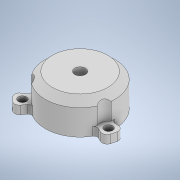
# Autodesk Inventor part: Knob
Saved by Autodesk Inventor 2022 (Build 260153000, 153)
## iProperties
Created: 2022-04-06
Part Number: Knob
Material: Generic
Document SubType Name: Modeling
Designer: awp
Density: 1 g/cm^3
Appearance: Default
Author: awp
Autodesk Inventor part; units mm, degrees
ref_plane "YZ Plane" through (0, 0, 0) normal (1, 0, 0) x (0, 1, 0)
ref_plane "XZ Plane" through (0, 0, 0) normal (0, 1, 0) x (-1, 0, 0)
ref_plane "XY Plane" through (0, 0, 0) normal (0, 0, 1) x (1, 0, 0)
sketch "Sketch1" plane through (0, 0, 0) normal (0, 1, 0) x (-1, 0, 0)
  circle A0 centre (0, 0) radius 2
  circle A1 centre (0, 0) radius 12.7
  dimension "d0" = 4
  dimension "d1" = 25.4
  constraints: 2 centre point, 2 coincident
  measures "d0" diameter of A0
  measures "d1" diameter of A1
extrude "Extrusion1" add sketch "Sketch1" along normal blind 3
sketch "Sketch3" plane through (0, 0, 0) normal (0, -1, 0) x (1, 0, 0)
  circle A0 centre (0, 0) radius 11.1125
  circle A1 centre (0, 0) radius 12.7 projected
  circle A2 centre (0, 0) radius 2 projected
  circle A3 centre (0, 0) radius 12.7 projected
  circle A4 centre (0, 0) radius 2 projected
  circle A5 centre (0, 0) radius 12.7
  dimension "d14" = 22.225
  constraints: 2 centre point, 2 coincident, 1 concentric
  measures "d14" diameter of A0
extrude "Extrusion3" add sketch "Sketch3" along normal blind 8.858 contours A1
sketch "Sketch4" plane through (0, 0, 0) normal (0, -1, 0) x (1, 0, 0)
  circle A0 centre (0, 0) radius 2 projected
  circle A1 centre (0, 0) radius 2 projected
  line L0 (-1.9732, -0.3262) -> (-3.4732, -0.3262)
  line L1 (-3.4732, -0.3262) -> (-1.9933, -0.3262)
  line L2 (-1.9933, -0.3262) -> (-1.9933, 7.2938)
  line L3 (-1.9933, 7.2938) -> (-3.4732, 7.2938)
  line L4 (-3.4732, 7.2938) -> (-3.4732, -0.3262)
  line L5 (-3.4732, 7.2938) -> (-4.7432, 7.2938)
  line L6 (-4.7432, 7.2938) -> (-4.7432, 3.4838)
  line L7 (-4.7432, 3.4838) -> (-3.4732, 3.4838)
  line L8 (-3.4732, 3.4838) -> (-3.4732, 7.2938)
  line L9 (-1.9933, 7.2938) -> (-0.7233, 7.2938)
  line L10 (-0.7233, 7.2938) -> (-0.7233, 3.4838)
  line L11 (-0.7233, 3.4838) -> (-1.9933, 3.4838)
  line L12 (-1.9933, 3.4838) -> (-1.9933, 7.2938)
  line L13 (-3.4732, -0.3262) -> (-1.9933, -0.3262)
  line L14 (-1.9933, -0.3262) -> (-1.9933, -7.3112)
  line L15 (-1.9933, -7.3112) -> (-3.4732, -7.3112)
  line L16 (-3.4732, -7.3112) -> (-3.4732, -0.3262)
  line L17 (-3.4732, -7.3112) -> (-4.7432, -7.3112)
  line L18 (-4.7432, -7.3112) -> (-4.7432, -3.5012)
  line L19 (-4.7432, -3.5012) -> (-3.4732, -3.5012)
  line L20 (-3.4732, -3.5012) -> (-3.4732, -7.3112)
  line L21 (-1.9933, -7.3112) -> (-0.7233, -7.3112)
  line L22 (-0.7233, -7.3112) -> (-0.7233, -3.5012)
  line L23 (-0.7233, -3.5012) -> (-1.9933, -3.5012)
  line L24 (-1.9933, -3.5012) -> (-1.9933, -7.3112)
  line L25 (-3.4732, -7.3112) -> (-4.7432, -6.0412)
  line L26 (-3.4732, -7.3112) -> (-1.6772, -7.3112) construction
  point P0 (-1.9933, 3.4838)
  point P1 (-3.4732, 3.4838)
  point P2 (-3.4732, -3.5012)
  point P3 (-1.9933, -3.5012)
  dimension "d17" = 1.5
  dimension "d18" = 7.62
  dimension "d19" = 1.27
  dimension "d20" = 3.81
  dimension "d21" = 1.27
  dimension "d22" = 3.81
  dimension "d37" = 6.985
  dimension "d38" = 1.27
  dimension "d39" = 3.81
  dimension "d40" = 1.27
  dimension "d41" = 135
  constraints: 54 end point, 12 parallel, 8 horizontal, 6 perpendicular, 2 point on line, 1 equal length, 2 other
  measures "d17" distance of L0.start L0.end
  measures "d18" distance of L2.end L1.end
  measures "d19" distance of L7.end L6.end
  measures "d20" distance of L6.end L5.end
  measures "d21" distance of L10.end L11.end
  measures "d22" distance of L9.end L10.end
  measures "d37" distance of L13.end L14.end
  measures "d38" distance of L18.end L19.end
  measures "d39" distance of L17.end L18.end
  measures "d40" distance of L23.end L22.end
  measures "d41" angle of L26 L25
extrude "Extrusion4" add sketch "Sketch4" along normal blind 2 contours L23 L22 L21 L14 | L16 L25 L18 L19
sketch "Sketch5" plane through (0, 3, 0) normal (0, 1, 0) x (1, 0, 0)
  circle A0 centre (0, 0) radius 12.7 projected
  circle A1 centre (0, 0) radius 2 projected
  circle A2 centre (0, 0) radius 12.7 projected
  line L0 (0, 12.7) -> (0, 14.605)
  line L1 (0, 14.605) -> (2.0758, 12.5292)
  line L2 (0, 14.605) -> (-2.0758, 12.5292)
  line L3 (0, 14.605) -> (2.9356, 14.605) construction
  line L4 (-4.5132, 13.8902) -> (-1.8975, 12.5574)
  line L5 (-3.9245, 12.0784) -> (-4.5132, 13.8902)
  line L6 (-4.5132, 13.8902) -> (-5.8459, 11.2745)
  line L7 (-8.5846, 11.8157) -> (-5.6851, 11.3565)
  line L8 (-7.4649, 10.2745) -> (-8.5846, 11.8157)
  line L9 (-8.5846, 11.8157) -> (-9.0438, 8.9162)
  line L10 (-11.8157, 8.5846) -> (-8.9162, 9.0438)
  line L11 (-10.2745, 7.4649) -> (-11.8157, 8.5846)
  line L12 (-11.8157, 8.5846) -> (-11.3565, 5.6851)
  line L13 (-13.8902, 4.5132) -> (-11.2745, 5.8459)
  line L14 (-12.0784, 3.9245) -> (-13.8902, 4.5132)
  line L15 (-13.8902, 4.5132) -> (-12.5574, 1.8975)
  line L16 (-14.605, 0) -> (-12.5292, 2.0758)
  line L17 (-12.7, 0) -> (-14.605, 0)
  line L18 (-14.605, 0) -> (-12.5292, -2.0758)
  line L19 (-13.8902, -4.5132) -> (-12.5574, -1.8975)
  line L20 (-12.0784, -3.9245) -> (-13.8902, -4.5132)
  line L21 (-13.8902, -4.5132) -> (-11.2745, -5.8459)
  line L22 (-11.8157, -8.5846) -> (-11.3565, -5.6851)
  line L23 (-10.2745, -7.4649) -> (-11.8157, -8.5846)
  line L24 (-11.8157, -8.5846) -> (-8.9162, -9.0438)
  line L25 (-8.5846, -11.8157) -> (-9.0438, -8.9162)
  line L26 (-7.4649, -10.2745) -> (-8.5846, -11.8157)
  line L27 (-8.5846, -11.8157) -> (-5.6851, -11.3565)
  line L28 (-4.5132, -13.8902) -> (-5.8459, -11.2745)
  line L29 (-3.9245, -12.0784) -> (-4.5132, -13.8902)
  line L30 (-4.5132, -13.8902) -> (-1.8975, -12.5574)
  line L31 (0, -14.605) -> (-2.0758, -12.5292)
  line L32 (0, -12.7) -> (0, -14.605)
  line L33 (0, -14.605) -> (2.0758, -12.5292)
  line L34 (4.5132, -13.8902) -> (1.8975, -12.5574)
  line L35 (3.9245, -12.0784) -> (4.5132, -13.8902)
  line L36 (4.5132, -13.8902) -> (5.8459, -11.2745)
  line L37 (8.5846, -11.8157) -> (5.6851, -11.3565)
  line L38 (7.4649, -10.2745) -> (8.5846, -11.8157)
  line L39 (8.5846, -11.8157) -> (9.0438, -8.9162)
  line L40 (11.8157, -8.5846) -> (8.9162, -9.0438)
  line L41 (10.2745, -7.4649) -> (11.8157, -8.5846)
  line L42 (11.8157, -8.5846) -> (11.3565, -5.6851)
  line L43 (13.8902, -4.5132) -> (11.2745, -5.8459)
  line L44 (12.0784, -3.9245) -> (13.8902, -4.5132)
  line L45 (13.8902, -4.5132) -> (12.5574, -1.8975)
  line L46 (14.605, 0) -> (12.5292, -2.0758)
  line L47 (12.7, 0) -> (14.605, 0)
  line L48 (14.605, 0) -> (12.5292, 2.0758)
  line L49 (13.8902, 4.5132) -> (12.5574, 1.8975)
  line L50 (12.0784, 3.9245) -> (13.8902, 4.5132)
  line L51 (13.8902, 4.5132) -> (11.2745, 5.8459)
  line L52 (11.8157, 8.5846) -> (11.3565, 5.6851)
  line L53 (10.2745, 7.4649) -> (11.8157, 8.5846)
  line L54 (11.8157, 8.5846) -> (8.9162, 9.0438)
  line L55 (8.5846, 11.8157) -> (9.0438, 8.9162)
  line L56 (7.4649, 10.2745) -> (8.5846, 11.8157)
  line L57 (8.5846, 11.8157) -> (5.6851, 11.3565)
  line L58 (4.5132, 13.8902) -> (5.8459, 11.2745)
  line L59 (3.9245, 12.0784) -> (4.5132, 13.8902)
  line L60 (4.5132, 13.8902) -> (1.8975, 12.5574)
  point P0 (-1.9969, 12.6081)
  point P1 (-5.7953, 11.3739)
  point P2 (-9.0264, 9.0264)
  point P3 (-11.3739, 5.7953)
  point P4 (-12.6081, 1.9969)
  point P5 (-12.6081, -1.9969)
  point P6 (-11.3739, -5.7953)
  point P7 (-9.0264, -9.0264)
  point P8 (-5.7953, -11.3739)
  point P9 (-1.9969, -12.6081)
  point P10 (1.9969, -12.6081)
  point P11 (5.7953, -11.3739)
  point P12 (9.0264, -9.0264)
  point P13 (11.3739, -5.7953)
  point P14 (12.6081, -1.9969)
  point P15 (12.6081, 1.9969)
  point P16 (11.3739, 5.7953)
  point P17 (9.0264, 9.0264)
  point P18 (5.7953, 11.3739)
  point P19 (1.9969, 12.6081)
  dimension "d28" = 1.905
  dimension "d29" = 45
  dimension "d30" = 135
  dimension "d33" = 360
  constraints: 122 end point, 2 point on circle, 1 equal length, 1 horizontal, 1 vertical, 143 other
  measures "d28" distance of L0.start L0.end
  measures "d29" angle of L0 L1
  measures "d30" angle of L2 L3
extrude "Extrusion5" [suppressed]
fillet "Fillet1" [suppressed]
sketch "Sketch8" plane through (0, -8.858, 0) normal (0, -1, 0) x (1, 0, 0)
  circle A0 centre (13.4621, 6.4384) radius 1.5 projected
  line L0 (16.2108, 4.5139) -> (12.5404, 3.4919) projected
  arc A1 (12.5404, 3.4919) -> (10.5899, 7.5704) centre (0, 0) ccw projected
  line L1 (10.5899, 7.5704) -> (13.6893, 9.7861) projected
  arc A2 (16.2108, 4.5139) -> (13.6893, 9.7861) centre (0, 0) ccw projected
  circle A3 centre (-12.3435, 8.3856) radius 1.5 projected
  line L2 (-12.0145, 11.782) -> (-9.2943, 9.1144) projected
  arc A4 (-9.2943, 9.1144) -> (-11.851, 5.3859) centre (0, 0) ccw projected
  line L3 (-11.851, 5.3859) -> (-15.3196, 6.9623) projected
  arc A5 (-12.0145, 11.782) -> (-15.3196, 6.9623) centre (0, 0) ccw projected
  circle A6 centre (-1.2201, -14.8725) radius 1.5 projected
  line L4 (-4.1963, -16.2959) -> (-3.2462, -12.6063) projected
  arc A7 (-3.2462, -12.6063) -> (1.2612, -12.9563) centre (0, 0) ccw projected
  line L5 (1.2612, -12.9563) -> (1.6303, -16.7483) projected
  arc A8 (-4.1963, -16.2959) -> (1.6303, -16.7483) centre (0, 0) ccw projected
  circle A9 centre (0, 0) radius 12.7 projected
  line L6 (-4.1963, -16.2959) -> (-3.167, -12.2988)
  line L7 (1.6303, -16.7483) -> (1.2304, -12.6403)
  line L8 (16.2108, 4.5139) -> (12.2346, 3.4067)
  line L9 (13.6893, 9.7861) -> (10.3316, 7.3857)
  line L10 (-12.0145, 11.782) -> (-9.0676, 8.8921)
  line L11 (-15.3196, 6.9623) -> (-11.562, 5.2545)
  point P0 (10.5899, 7.5704)
  point P1 (-11.851, 5.3859)
  point P2 (1.2612, -12.9563)
  constraints: 12 end point, 6 point on circle, 2 point on line
extrude "Extrusion6" [suppressed]
fillet "Fillet2" [suppressed]
chamfer "Chamfer2" distance 2.54 angle 45 1 edges at (12.7, 3, 0)
sketch "Sketch9" plane through (0, 0, 0) normal (0, -1, 0) x (1, 0, 0)
  circle A0 centre (0, 0) radius 3
  circle A1 centre (0, 0) radius 4
  line L0 (-0.7233, -3.5012) -> (-1.9933, -3.5012) projected
  line L1 (-1.9933, -3.5012) -> (-1.9933, -7.3112) projected
  line L2 (-1.9933, -7.3112) -> (-0.7233, -7.3112) projected
  line L3 (-0.7233, -7.3112) -> (-0.7233, -3.5012) projected
  line L4 (-3.4732, -7.3112) -> (-3.4732, -3.5012) projected
  line L5 (-3.4732, -3.5012) -> (-4.7432, -3.5012) projected
  line L6 (-4.7432, -3.5012) -> (-4.7432, -6.0412) projected
  line L7 (-4.7432, -6.0412) -> (-3.4732, -7.3112) projected
  line L8 (-1.9933, -3.5012) -> (-1.9062, -2.3166)
  line L9 (-3.4732, -3.5012) -> (-4.7432, -3.5012) projected
  line L10 (-3.4732, -3.5012) -> (-3, 0)
  point P0 (-3.3046, -2.2538)
  point P1 (-1.991, -3.4693)
  dimension "d49" = 6
  dimension "d50" = 8
  constraints: 4 end point, 2 centre point, 2 coincident, 2 point on circle
  measures "d49" diameter of A0
  measures "d50" diameter of A1
extrude "Extrusion7" add sketch "Sketch9" along normal blind 6.35 contours A0 L10 A1 L3 L0 L8 | L0 L3 A1
sketch "Sketch10" plane through (0, 3, 0) normal (0, 1, 0) x (1, 0, 0)
  circle A0 centre (-12.3435, -8.3856) radius 1.5 projected
  circle A1 centre (-1.2201, 14.8725) radius 1.5 projected
  circle A2 centre (13.4621, -6.4384) radius 1.5 projected
  circle A3 centre (-12.3435, -8.3856) radius 3.175
  circle A4 centre (-1.2201, 14.8725) radius 3.175
  circle A5 centre (13.4621, -6.4384) radius 3.175
  point P0 (0, 0)
  dimension "d53" = 6.35
  dimension "d54" = 6.35
  dimension "d55" = 6.35
  constraints: 3 centre point, 3 coincident
  measures "d53" diameter of A3
  measures "d54" diameter of A4
  measures "d55" diameter of A5
extrude "Extrusion8" [suppressed]
fillet "Fillet3" [suppressed]
thicken "Thicken3" [suppressed]
thicken "Thicken4" [suppressed]
thicken "Thicken5" [suppressed]
sketch "Sketch11" plane through (0, 0, 0) normal (0, -1, 0) x (1, 0, 0)
  arc A0 (-0.7233, -3.9341) -> (-3.3046, -2.2538) centre (0, 0) ccw projected
  line L0 (-0.7233, -3.9341) -> (-0.7233, -7.3112) projected
  line L1 (-0.7233, -7.3112) -> (-1.9933, -7.3112) projected
  line L2 (-1.9933, -7.3112) -> (-1.9933, -3.5012) projected
  line L3 (-1.9933, -3.5012) -> (-1.9343, -3.5012) projected
  arc A1 (-1.991, -3.4693) -> (-1.9343, -3.5012) centre (0, 0) ccw projected
  line L4 (-1.991, -3.4693) -> (-1.9062, -2.3166) projected
  arc A2 (-1.9062, -2.3166) -> (-3, 0) centre (0, 0) ccw projected
  line L5 (-3, 0) -> (-3.3046, -2.2538) projected
  line L6 (-3.4732, -7.3112) -> (-4.7432, -6.0412) projected
  line L7 (-4.7432, -6.0412) -> (-4.7432, -3.5012) projected
  line L8 (-4.7432, -3.5012) -> (-3.4732, -3.5012) projected
  line L9 (-3.4732, -3.5012) -> (-3.4732, -7.3112) projected
  circle A3 centre (0, 0) radius 11.1125 projected
  circle A4 centre (0, 0) radius 2 projected
  line L10 (-3.3046, -2.2538) -> (-3.4732, -3.5012)
  line L11 (-1.9933, -7.3112) -> (-1.9933, -3.5012) projected
  line L12 (-1.9933, -7.3112) -> (-1.9933, -10.9323)
  line L13 (-3.4732, -7.3112) -> (-4.7432, -6.0412) projected
  line L14 (-3.4732, -7.3112) -> (-3.4732, -10.5558)
  circle A5 centre (0, 0) radius 11.1125 projected
  constraints: 6 end point, 1 collinear, 1 parallel, 1 point on circle, 2 other
extrude "Extrusion9" add sketch "Sketch11" along normal up to surface (2 mm away) contours A0 L10 L8 L7 L6 L14 A3 L12 L1 L0
sketch "Sketch12" plane through (0, -8.858, 0) normal (0, -1, 0) x (1, 0, 0)
  circle A0 centre (0, 0) radius 12.7 projected
  circle A1 centre (0, 0) radius 11.1125 projected
  arc A2 (15.5202, 1.4015) -> (17.1016, 3.5319) centre (15.3603, 3.1723) ccw
  arc A3 (17.1016, 3.5319) -> (16.5455, 5.5845) centre (0, 0) ccw
  arc A4 (16.5455, 5.5845) -> (14.1049, 6.6252) centre (14.8608, 5.0159) ccw
  line L0 (14.1049, 6.6252) -> (12.5922, 5.9147)
  arc A5 (10.9566, 6.422) -> (12.5922, 5.9147) centre (12.0523, 7.0642) ccw
  arc A6 (10.9566, 6.422) -> (-6.3392, 11.0047) centre (0, 0) ccw
  arc A7 (-8.0114, 11.3739) -> (-6.3392, 11.0047) centre (-6.9731, 12.1052) ccw
  line L1 (-8.0114, 11.3739) -> (-8.9738, 12.7402)
  arc A8 (-8.9738, 12.7402) -> (-11.6095, 13.0445) centre (-10.4274, 11.7163) ccw
  arc A9 (-11.6095, 13.0445) -> (-13.109, 11.5366) centre (0, 0) ccw
  arc A10 (-13.109, 11.5366) -> (-12.7901, 8.9026) centre (-11.7743, 10.3619) ccw
  line L2 (-12.7901, 8.9026) -> (-11.4184, 7.9479)
  arc A11 (-11.0399, 6.2777) -> (-11.4184, 7.9479) centre (-12.1439, 6.9055) ccw
  arc A12 (-11.0399, 6.2777) -> (-6.3608, -10.9923) centre (0, 0) ccw
  arc A13 (-5.8443, -12.625) -> (-6.3608, -10.9923) centre (-6.9968, -12.0915) ccw
  line L3 (-5.8443, -12.625) -> (-6.5464, -14.1417)
  arc A14 (-6.5464, -14.1417) -> (-5.4921, -16.5764) centre (-4.9329, -14.8886) ccw
  arc A15 (-5.4921, -16.5764) -> (-3.4364, -17.121) centre (0, 0) ccw
  arc A16 (-3.4364, -17.121) -> (-1.3149, -15.5278) centre (-3.0865, -15.3778) ccw
  line L4 (-1.3149, -15.5278) -> (-1.1739, -13.8625)
  arc A17 (0.0833, -12.6997) -> (-1.1739, -13.8625) centre (0.0916, -13.9697) ccw
  arc A18 (0.0833, -12.6997) -> (12.7, -0.0124) centre (0, 0) ccw
  arc A19 (13.8558, 1.2512) -> (12.7, -0.0124) centre (13.97, -0.0137) ccw
  line L5 (13.8558, 1.2512) -> (15.5202, 1.4015)
  circle A20 centre (-3.822, -14.4247) radius 1.5
  circle A21 centre (14.3861, 3.9652) radius 1.5
  circle A22 centre (-10.5352, 10.5684) radius 1.5
  circle A23 centre (0, 0) radius 11.1125
  point P0 (10.9566, 6.422)
  point P1 (12.7, -0.0124)
  point P2 (-11.0399, 6.2777)
  point P3 (-6.3392, 11.0047)
  point P4 (0.0833, -12.6997)
  point P5 (-6.3608, -10.9923)
  constraints: 36 point on circle, 22 centre point, 12 end point
extrude "Extrusion10" add sketch "Sketch12" against normal blind 3.048 contours A0 A5 L0 A4 A3 A2 L5 A19 | A0 A11 L2 A10 A9 A8 L1 A7 | A17 L4 A16 A15 A14 L3 A13 A0
sketch "Sketch13" plane through (0, -5.81, 0) normal (0, 1, 0) x (1, 0, 0)
  arc A0 (12.5922, -5.9147) -> (10.9566, -6.422) centre (12.0523, -7.0642) ccw projected
  line L0 (12.5922, -5.9147) -> (14.1049, -6.6252) projected
  arc A1 (14.1049, -6.6252) -> (16.5455, -5.5845) centre (14.8608, -5.0159) ccw projected
  arc A2 (16.5455, -5.5845) -> (17.1016, -3.5319) centre (0, 0) ccw projected
  arc A3 (17.1016, -3.5319) -> (15.5202, -1.4015) centre (15.3603, -3.1723) ccw projected
  line L1 (15.5202, -1.4015) -> (13.8558, -1.2512) projected
  arc A4 (12.7, 0.0124) -> (13.8558, -1.2512) centre (13.97, 0.0137) ccw projected
  arc A5 (10.9566, -6.422) -> (12.7, 0.0124) centre (0, 0) ccw projected
  circle A6 centre (14.3861, -3.9652) radius 1.5 projected
  arc A7 (-11.4184, -7.9479) -> (-11.0399, -6.2777) centre (-12.1439, -6.9055) ccw projected
  line L2 (-11.4184, -7.9479) -> (-12.7901, -8.9026) projected
  arc A8 (-12.7901, -8.9026) -> (-13.109, -11.5366) centre (-11.7743, -10.3619) ccw projected
  arc A9 (-13.109, -11.5366) -> (-11.6095, -13.0445) centre (0, 0) ccw projected
  arc A10 (-11.6095, -13.0445) -> (-8.9738, -12.7402) centre (-10.4274, -11.7163) ccw projected
  line L3 (-8.9738, -12.7402) -> (-8.0114, -11.3739) projected
  arc A11 (-6.3392, -11.0047) -> (-8.0114, -11.3739) centre (-6.9731, -12.1052) ccw projected
  arc A12 (-11.0399, -6.2777) -> (-6.3392, -11.0047) centre (0, 0) ccw projected
  circle A13 centre (-10.5352, -10.5684) radius 1.5 projected
  arc A14 (-1.1739, 13.8625) -> (0.0833, 12.6997) centre (0.0916, 13.9697) ccw projected
  line L4 (-1.1739, 13.8625) -> (-1.3149, 15.5278) projected
  arc A15 (-1.3149, 15.5278) -> (-3.4364, 17.121) centre (-3.0865, 15.3778) ccw projected
  arc A16 (-3.4364, 17.121) -> (-5.4921, 16.5764) centre (0, 0) ccw projected
  arc A17 (-5.4921, 16.5764) -> (-6.5464, 14.1417) centre (-4.9329, 14.8886) ccw projected
  line L5 (-6.5464, 14.1417) -> (-5.8443, 12.625) projected
  arc A18 (-6.3608, 10.9923) -> (-5.8443, 12.625) centre (-6.9968, 12.0915) ccw projected
  arc A19 (0.0833, 12.6997) -> (-6.3608, 10.9923) centre (0, 0) ccw projected
  circle A20 centre (-3.822, 14.4247) radius 1.5 projected
  circle A21 centre (14.3861, -3.9652) radius 3.175
  circle A22 centre (-10.5352, -10.5684) radius 3.175
  circle A23 centre (-3.822, 14.4247) radius 3.175
  dimension "d69" = 6.35
  dimension "d70" = 6.35
  dimension "d71" = 6.35
  constraints: 3 centre point, 3 coincident
  measures "d69" diameter of A21
  measures "d70" diameter of A22
  measures "d71" diameter of A23
extrude "Extrusion11" cut sketch "Sketch13" along normal up to surface (8.81 mm away) contours L0 A1 A2 A3 L1 A4 A21 A0 | A0 A21 A5 A4 L1 A3 A2 A1 L0 | A21 A5 | A6 | L2 A8 A9 A10 L3 A11 A22 A7 | A7 A22 A12 A11 L3 A10 A9 A8 L2 | A22 A12 | A13 | L4 A15 A16 A17 L5 A18 A23 A14 | A14 A23 A19 A18 L5 A17 A16 A15 L4 | A23 A19 | A20
body "Solid1"
